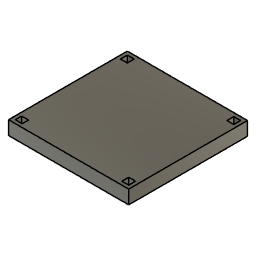
2D lidar v1 (1) (Autodesk Fusion 360 design; units mm, degrees)
Autodesk Fusion 360 part; units mm, degrees
sketch "Sketch1" plane through (0, 0, 0) normal (0, 0, 1) x (1, 0, 0)
  line L0 (0, 0) -> (44, 0)
  line L1 (44, 0) -> (44, 43.5)
  line L2 (44, 43.5) -> (0, 43.5)
  line L3 (0, 43.5) -> (0, 0)
  dimension "d1" = 44
  dimension "d2" = 43.5
  constraint horizontal L0
  constraint vertical L1
  constraint horizontal L2
  constraint vertical L3
  constraint coincident L0.start L3.end
  measures "d1" distance of L0.start L0.end
  measures "d2" distance of L0.start L2.end
extrude "Extrude1" add sketch "Sketch1" along normal blind 5
sketch "Sketch2" plane through (0, 0, 5) normal (0, 0, 1) x (-1, 0, 0)
  line L0 (0, -43.5) -> (0, 0)
  line L1 (0, 0) -> (-44, 0)
  line L2 (-44, 0) -> (-44, -43.5)
  line L3 (-44, -43.5) -> (0, -43.5)
  line L4 (0, 0) -> (0, -1.25)
  line L5 (0, -1.25) -> (-1.25, -1.25)
  line L6 (-1.25, -1.25) -> (-3.75, -1.25)
  line L7 (-3.75, -1.25) -> (-3.75, -3.541)
  line L8 (-3.75, -3.541) -> (-1.25, -3.541)
  line L9 (-1.25, -3.541) -> (-1.25, -1.25)
  line L10 (-44, 0) -> (-42.75, 0)
  line L11 (-42.75, 0) -> (-42.75, -1.25)
  line L12 (-42.75, -1.25) -> (-40.25, -1.25)
  line L13 (-40.25, -1.25) -> (-40.25, -3.75)
  line L14 (-40.25, -3.75) -> (-42.75, -3.75)
  line L15 (-42.75, -3.75) -> (-42.75, -1.25)
  line L16 (0, -43.5) -> (-1.25, -43.5)
  line L17 (-1.25, -43.5) -> (-1.25, -42.25)
  line L18 (-1.25, -42.25) -> (-3.75, -42.25)
  line L19 (-3.75, -42.25) -> (-3.75, -39.75)
  line L20 (-3.75, -39.75) -> (-1.25, -39.75)
  line L21 (-1.25, -39.75) -> (-1.25, -42.25)
  line L22 (-44, -43.5) -> (-42.75, -43.5)
  line L23 (-42.75, -43.5) -> (-42.75, -42.25)
  line L24 (-42.75, -42.25) -> (-40.25, -42.25)
  line L25 (-40.25, -42.25) -> (-40.25, -39.75)
  line L26 (-40.25, -39.75) -> (-42.75, -39.75)
  line L27 (-42.75, -39.75) -> (-42.75, -42.25)
  dimension "d5" = 1.25
  dimension "d6" = 1.25
  dimension "d7" = 2.5
  dimension "d8" = 1.25
  dimension "d9" = 1.25
  dimension "d10" = 2.5
  dimension "d11" = 2.5
  dimension "d12" = 1.25
  dimension "d13" = 1.25
  dimension "d14" = 2.5
  dimension "d15" = 2.5
  dimension "d16" = 1.25
  dimension "d17" = 1.25
  dimension "d18" = 2.5
  dimension "d19" = 2.5
  constraint coincident L0.end L1.start
  constraint perpendicular L1 L4
  constraint perpendicular L4 L5
  constraint horizontal L6
  constraint vertical L7
  constraint horizontal L8
  constraint vertical L9
  constraint coincident L1.end L2.start
  constraint perpendicular L2 L10
  constraint perpendicular L10 L11
  constraint horizontal L12
  constraint vertical L13
  constraint horizontal L14
  constraint vertical L15
  constraint coincident L0.start L3.end
  constraint perpendicular L0 L16
  constraint perpendicular L16 L17
  constraint horizontal L18
  constraint vertical L19
  constraint horizontal L20
  constraint vertical L21
  constraint coincident L2.end L3.start
  constraint perpendicular L2 L22
  constraint perpendicular L22 L23
  constraint horizontal L24
  constraint vertical L25
  constraint horizontal L26
  constraint vertical L27
  measures "d5" distance of L0.end L4.end
  measures "d6" distance of L4.end L5.end
  measures "d7" distance of L5.end L6.end
  measures "d8" distance of L1.end L10.end
  measures "d9" distance of L10.end L11.end
  measures "d10" distance of L11.end L12.end
  measures "d11" distance of L11.end L14.end
  measures "d12" distance of L0.start L16.end
  measures "d13" distance of L16.end L17.end
  measures "d14" distance of L17.end L18.end
  measures "d15" distance of L17.end L20.end
  measures "d16" distance of L2.end L22.end
  measures "d17" distance of L22.end L23.end
  measures "d18" distance of L23.end L24.end
  measures "d19" distance of L23.end L26.end
extrude "Extrude2" cut sketch "Sketch2" against normal blind 1000 contours L6 L7 L8 L9 | L12 L13 L14 L15 | L18 L19 L20 L21 | L24 L25 L26 L27
